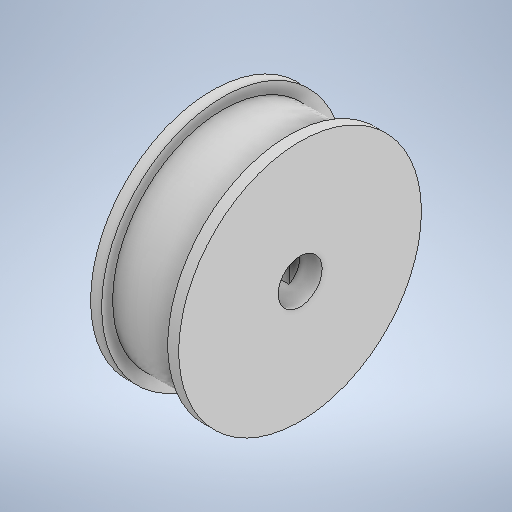
# Autodesk Inventor part: RODA MOTOR-PASSO
Saved by Autodesk Inventor 2025.2 (Build 292293000, 293)
## iProperties
Created: 2025-05-13
Part Number: RODA MOTOR-PASSO
Material: Genérico
Document SubType Name: Modeling
Designer: marce
Density: 1 g/cm^3
Appearance: Padrão
Author: marce
Autodesk Inventor part; units mm, degrees
ref_plane "YZ Plane" through (0, 0, 0) normal (1, 0, 0) x (0, 1, 0)
ref_plane "XZ Plane" through (0, 0, 0) normal (0, 1, 0) x (-1, 0, 0)
ref_plane "XY Plane" through (0, 0, 0) normal (0, 0, 1) x (1, 0, 0)
sketch "Esboço1" plane through (0, 0, 0) normal (1, 0, 0) x (0, 1, 0)
  circle A0 centre (0, 0) radius 10
  dimension "d0" = 20
  constraints: 1 centre point, 1 coincident
  measures "d0" diameter of A0
extrude "Extrusão1" add sketch "Esboço1" along normal blind 8
sketch "Esboço2" plane through (8, 0, 0) normal (1, 0, 0) x (0, 0, -1)
  circle A0 centre (0, 0) radius 2
  dimension "d3" = 4
  constraints: 1 centre point, 1 coincident
  measures "d3" diameter of A0
extrude "Extrusão2" cut sketch "Esboço2" against normal blind 2
sketch "Esboço3" plane through (6, 0, 0) normal (1, 0, 0) x (0, 0, -1)
  line L0 (1, 0) -> (1, 1.7321)
  circle A0 centre (0, 0) radius 2 projected
  line L1 (1, 0) -> (1, -1.7321)
  line L2 (-1, 0) -> (-1, 1.7321)
  line L3 (-1, 0) -> (-1, -1.7321)
  arc A1 (-1, 1.7321) -> (0, 2) centre (0, 0) ccw
  arc A2 (-1, -1.7321) -> (1, -1.7321) centre (0, 0) ccw
  dimension "d6" = 1
  dimension "d7" = 1
  constraints: 12 point on circle, 8 end point, 2 centre point, 2 concentric, 2 vertical, 1 point on line
  measures "d6" distance of point (0, 0) L2.start
  measures "d7" distance of point (0, 0) L0.start
extrude "Extrusão3" cut sketch "Esboço3" against normal through all contours L1 A0 L3 L2 L0
sketch "Esboço4" plane through (8, 0, 0) normal (1, 0, 0) x (0, 0, -1)
  circle A0 centre (0, 0) radius 2
  circle A1 centre (0, 0) radius 11
  dimension "d10" = 22
  constraints: 2 centre point, 2 coincident
  measures "d10" diameter of A1
extrude "Extrusão4" add sketch "Esboço4" against normal blind 1
sketch "Esboço5" plane through (0, 0, 0) normal (-1, 0, 0) x (0, 0, 1)
  circle A0 centre (0, 0) radius 2
  circle A1 centre (0, 0) radius 11
  constraints: 2 centre point, 2 coincident
extrude "Extrusão5" add sketch "Esboço5" against normal blind 1
